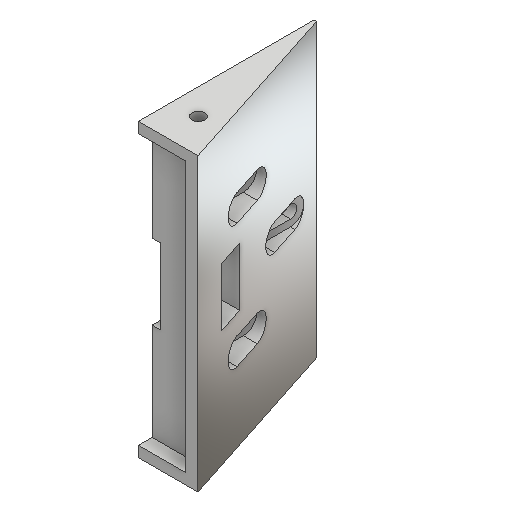
# Autodesk Inventor part: 3DP_PLA_Front_plow
Saved by Autodesk Inventor 2026.1 (Build 301233000, 233)
## iProperties
Created: 2016-05-01
Part Number: 3DP_PLA_Front_plow
Material: Ogólny
Document SubType Name: Modeling
Designer: Andrzej
Density: 1 g/cm^3
Appearance: Domyślna
Mass: 15.1974 g
Surface Area: 84.5843 cm^2
Volume: 15.1974 cm^3
Author: Andrzej
Autodesk Inventor part; units mm, degrees
ref_plane "YZ Plane" through (0, 0, 0) normal (1, 0, 0) x (0, 1, 0)
ref_plane "XZ Plane" through (0, 0, 0) normal (0, 1, 0) x (-1, 0, 0)
ref_plane "XY Plane" through (0, 0, 0) normal (0, 0, 1) x (1, 0, 0)
sketch "Szkic1" plane through (0, 0, 0) normal (0, 0, 1) x (1, 0, 0)
  line L0 (-7.2343, -6.8907) -> (6.6657, -6.8907)
  line L1 (-7.2343, -6.8907) -> (-7.2343, 34.1093)
  line L2 (-7.2343, 34.1093) -> (-6.6343, 34.1093)
  line L3 (-6.6343, 34.1093) -> (6.6657, -6.8907)
  point P0 (0, 0)
  dimension "d0" = 13.9
  dimension "d1" = 41
  dimension "d2" = 0.6
  constraints: 8 end point, 2 horizontal, 1 vertical
  measures "d0" distance of L0.start L0.end
  measures "d1" distance of L0.start L1.end
  measures "d2" distance of L1.end L2.end
extrude "Wyciągnięcie proste1" add sketch "Szkic1" along normal blind 68
sketch "Szkic2" plane through (-7.2343, -6.8907, 0) normal (-1, 0, 0) x (0, 0, 1)
  line L0 (0, 41) -> (0, 0) projected
  line L1 (0, 0) -> (68, 0) projected
  line L2 (68, 41) -> (68, 0) projected
  line L3 (0, 41) -> (68, 41) projected
  line L4 (68, 17.5) -> (68, 0)
  line L5 (53.5, 17.5) -> (68, 17.5)
  line L6 (53.5, 17.5) -> (53.5, 47.1186)
  line L7 (0, 47.1186) -> (53.5, 47.1186)
  line L8 (0, 0) -> (0, 47.1186)
  line L9 (68, 0) -> (0, 0)
  line L10 (68, 0) -> (0, 0)
  line L11 (14.5, 0) -> (14.5, 47.1186)
  line L12 (0, 47.1186) -> (53.5, 47.1186)
  line L13 (14.5, 12) -> (39.4786, 12)
  line L14 (19.5, 13.5) -> (19.5, 20.5) construction
  line L15 (21, 13.5) -> (21, 20.5)
  line L16 (18, 20.5) -> (18, 13.5)
  arc A0 (18, 13.5) -> (21, 13.5) centre (19.5, 13.5) ccw
  arc A1 (21, 20.5) -> (18, 20.5) centre (19.5, 20.5) ccw
  line L17 (48.5, 13.5) -> (48.5, 20.5) construction
  line L18 (50, 13.5) -> (50, 20.5)
  line L19 (47, 20.5) -> (47, 13.5)
  arc A2 (47, 13.5) -> (50, 13.5) centre (48.5, 13.5) ccw
  arc A3 (50, 20.5) -> (47, 20.5) centre (48.5, 20.5) ccw
  line L20 (34, 26.5) -> (34, 33.5) construction
  line L21 (35.5, 26.5) -> (35.5, 33.5)
  line L22 (32.5, 33.5) -> (32.5, 26.5)
  arc A4 (32.5, 26.5) -> (35.5, 26.5) centre (34, 26.5) ccw
  arc A5 (35.5, 33.5) -> (32.5, 33.5) centre (34, 33.5) ccw
  point P0 (0, 6.8907)
  point P1 (82.8727, 0)
  point P2 (19.5, 17)
  point P3 (48.5, 17)
  point P4 (34, 30)
  dimension "d5" = 14.5
  dimension "d6" = 14.5
  dimension "d7" = 12
  dimension "d8" = 5
  dimension "d9" = 5
  dimension "d10" = 5
  dimension "d11" = 5
  dimension "d12" = 18
  dimension "d13" = 19.5
  dimension "d14" = 39
  dimension "d15" = 0
  dimension "d16" = 3.5
  dimension "d17" = 3
  dimension "d18" = 3
  dimension "d19" = 3.5
  dimension "d20" = 3
  constraints: 44 end point, 12 point on circle, 12 tangent, 6 centre point, 5 parallel, 3 midpoint, 3 point on line, 1 horizontal, 1 perpendicular, 1 vertical
  measures "d5" distance between parallel lines of L4 L6
  measures "d6" distance between parallel lines of L8 L11
  measures "d7" distance between parallel lines of L9 L13
  measures "d8" distance from line of L13 point (19.5, 17)
  measures "d9" distance from line of L11 point (19.5, 17)
  measures "d10" distance from line of L13 point (48.5, 17)
  measures "d11" distance from line of L6 point (48.5, 17)
  measures "d12" distance from line of L13 point (34, 30)
  measures "d13" distance from line of L11 point (34, 30)
  measures "d14" distance between parallel lines of L11 L6
  measures "d15" distance between parallel lines of L1 L9
  measures "d16" distance of point (19.5, 17) L14.end
  measures "d17" diameter of A1
  measures "d18" diameter of A3
  measures "d19" distance of point (34, 30) L20.end
  measures "d20" diameter of A5
extrude "Wyciągnięcie proste2" cut sketch "Szkic2" against normal blind 10 contours A0 L16 A1 L15 | A2 L19 A3 L18 | A4 L22 A5 L21
ref_plane "Płaszczyzna konstrukcyjna1" through (4.7657, -6.8907, 0) normal (-1, 0, 0) x (0, 0, 1)
sketch "Szkic3" plane through (4.7657, -6.8907, 0) normal (-1, 0, 0) x (0, 0, 1)
  arc A0 (50, 20.5) -> (47, 20.5) centre (48.5, 20.5) ccw projected
  line L0 (47, 20.5) -> (47, 13.5) projected
  arc A1 (48.7592, 12.0226) -> (50, 13.5) centre (48.5, 13.5) ccw projected
  line L1 (50, 13.5) -> (50, 20.5) projected
  arc A2 (21, 20.5) -> (18, 20.5) centre (19.5, 20.5) ccw projected
  line L2 (18, 20.5) -> (18, 13.5) projected
  arc A3 (19.7592, 12.0226) -> (21, 13.5) centre (19.5, 13.5) ccw projected
  line L3 (21, 13.5) -> (21, 20.5) projected
  arc A4 (35.5, 33.5) -> (32.5, 33.5) centre (34, 33.5) ccw projected
  line L4 (32.5, 33.5) -> (32.5, 26.5) projected
  arc A5 (32.5, 26.5) -> (35.5, 26.5) centre (34, 26.5) ccw projected
  line L5 (35.5, 26.5) -> (35.5, 33.5) projected
  line L6 (0, 0) -> (0, 41) projected
  line L7 (0, 41) -> (68, 41) projected
  line L8 (68, 0) -> (68, 41) projected
  line L9 (0, 0) -> (68, 0) projected
  line L10 (16.4, 13.5) -> (16.4, 20.5)
  arc A6 (22.6, 20.5) -> (16.4, 20.5) centre (19.5, 20.5) ccw
  line L11 (22.6, 20.5) -> (22.6, 13.5)
  arc A7 (16.4, 13.5) -> (22.6, 13.5) centre (19.5, 13.5) ccw
  arc A8 (30.9, 26.5) -> (37.1, 26.5) centre (34, 26.5) ccw
  line L12 (30.9, 26.5) -> (30.9, 33.5)
  arc A9 (37.1, 33.5) -> (30.9, 33.5) centre (34, 33.5) ccw
  line L13 (37.1, 33.5) -> (37.1, 26.5)
  line L14 (45.4, 13.5) -> (45.4, 20.5)
  arc A10 (51.6, 20.5) -> (45.4, 20.5) centre (48.5, 20.5) ccw
  line L15 (51.6, 20.5) -> (51.6, 13.5)
  arc A11 (45.4, 13.5) -> (51.6, 13.5) centre (48.5, 13.5) ccw
  arc A12 (47, 13.5) -> (48.2408, 12.0226) centre (48.5, 13.5) ccw projected
  line L16 (48.2408, 12.0226) -> (48.7592, 12.0226) projected
  arc A13 (18, 13.5) -> (19.2408, 12.0226) centre (19.5, 13.5) ccw projected
  line L17 (19.2408, 12.0226) -> (19.7592, 12.0226) projected
  point P0 (0, 6.8907)
  dimension "d24" = 1.6
  dimension "d25" = 1.6
  dimension "d26" = 1.6
  constraints: 12 end point, 12 point on circle, 6 centre point, 9 other
  measures "d24" distance between parallel lines of L2 L10
  measures "d25" radial gap between concentric circles of A5 A8
  measures "d26" distance between parallel lines of L0 L14
extrude "Wyciągnięcie proste3" cut sketch "Szkic3" along normal blind 8 contours L10 A6 L11 A7 | L14 A10 L15 A11
extrude "Wyciągnięcie proste4" cut sketch "Szkic3" along normal blind 10 contours L12 A9 L13 A8
sketch "Szkic4" plane through (-7.2343, -6.8907, 0) normal (0, -1, 0) x (1, 0, 0)
  line L0 (0, 0) -> (13.9, 0) projected
  line L1 (13.9, 0) -> (13.9, 68) projected
  line L2 (0, 68) -> (13.9, 68) projected
  line L3 (0, 0) -> (0, 68) projected
  line L4 (0, 0) -> (0, 68) projected
  line L5 (0, 65.5) -> (10.9, 65.5)
  line L6 (10.9, 65.5) -> (10.9, 2.5)
  line L7 (10.9, 2.5) -> (0, 2.5)
  point P0 (7.2343, 0)
  dimension "d31" = 2.5
  dimension "d32" = 3
  dimension "d33" = 2.5
  constraints: 6 end point, 3 perpendicular, 2 point on line
  measures "d31" distance between parallel lines of L2 L5
  measures "d32" distance between parallel lines of L1 L6
  measures "d33" distance between parallel lines of L0 L7
extrude "Wyciągnięcie proste5" cut sketch "Szkic4" against normal blind 3.2 contours L3 L5 L6 L7
sketch "Szkic5" plane through (-7.2343, -6.8907, 0) normal (-1, 0, 0) x (0, 0, 1)
  line L0 (2.5, 0) -> (2.5, 3.2) projected
  line L1 (2.5, 3.2) -> (65.5, 3.2) projected
  line L2 (65.5, 3.2) -> (65.5, 0) projected
  line L3 (65.5, 0) -> (68, 0) projected
  line L4 (68, 41) -> (68, 0) projected
  line L5 (0, 41) -> (68, 41) projected
  line L6 (0, 41) -> (0, 0) projected
  line L7 (0, 0) -> (2.5, 0) projected
  arc A0 (35.5, 33.5) -> (32.5, 33.5) centre (34, 33.5) ccw projected
  line L8 (35.5, 33.5) -> (35.5, 26.5) projected
  arc A1 (32.5, 26.5) -> (35.5, 26.5) centre (34, 26.5) ccw projected
  line L9 (32.5, 26.5) -> (32.5, 33.5) projected
  arc A2 (21, 20.5) -> (18, 20.5) centre (19.5, 20.5) ccw projected
  line L10 (21, 20.5) -> (21, 13.5) projected
  arc A3 (18, 13.5) -> (21, 13.5) centre (19.5, 13.5) ccw projected
  line L11 (18, 13.5) -> (18, 20.5) projected
  arc A4 (50, 20.5) -> (47, 20.5) centre (48.5, 20.5) ccw projected
  line L12 (50, 20.5) -> (50, 13.5) projected
  arc A5 (47, 13.5) -> (50, 13.5) centre (48.5, 13.5) ccw projected
  line L13 (47, 13.5) -> (47, 20.5) projected
  line L14 (65.5, 3.2) -> (2.5, 3.2) projected
  line L15 (29, 3.2) -> (39, 3.2)
  line L16 (39, 3.2) -> (39, 21.2)
  line L17 (39, 21.2) -> (29, 21.2)
  line L18 (29, 21.2) -> (29, 3.2)
  line L19 (2.5, 3.2) -> (65.5, 3.2) projected
  point P0 (0, 6.8907)
  dimension "d36" = 68
  dimension "d37" = 10
  dimension "d38" = 29
  dimension "d39" = 18
  constraints: 8 end point, 2 parallel, 1 horizontal, 1 perpendicular, 1 point on line
  measures "d36" distance of L5.start L4.start
  measures "d37" distance between parallel lines of L16 L18
  measures "d38" distance between parallel lines of L6 L18
  measures "d39" distance between parallel lines of L1 L17
extrude "Wyciągnięcie proste6" cut sketch "Szkic5" against normal blind 2 contours L18 L17 L16 L1
sketch "Szkic6" plane through (-7.2343, -6.8907, 0) normal (-1, 0, 0) x (0, 0, 1)
  line L0 (39, 21.2) -> (39, 3.2) projected
  line L1 (39, 3.2) -> (65.5, 3.2) projected
  line L2 (65.5, 3.2) -> (65.5, 0) projected
  line L3 (65.5, 0) -> (68, 0) projected
  line L4 (68, 41) -> (68, 0) projected
  line L5 (0, 41) -> (68, 41) projected
  line L6 (0, 41) -> (0, 0) projected
  line L7 (0, 0) -> (2.5, 0) projected
  line L8 (2.5, 0) -> (2.5, 3.2) projected
  line L9 (2.5, 3.2) -> (29, 3.2) projected
  line L10 (29, 3.2) -> (29, 21.2) projected
  line L11 (29, 21.2) -> (39, 21.2) projected
  arc A0 (35.5, 33.5) -> (32.5, 33.5) centre (34, 33.5) ccw projected
  line L12 (35.5, 33.5) -> (35.5, 26.5) projected
  arc A1 (32.5, 26.5) -> (35.5, 26.5) centre (34, 26.5) ccw projected
  line L13 (32.5, 26.5) -> (32.5, 33.5) projected
  arc A2 (21, 20.5) -> (18, 20.5) centre (19.5, 20.5) ccw projected
  line L14 (21, 20.5) -> (21, 13.5) projected
  arc A3 (18, 13.5) -> (21, 13.5) centre (19.5, 13.5) ccw projected
  line L15 (18, 13.5) -> (18, 20.5) projected
  arc A4 (50, 20.5) -> (47, 20.5) centre (48.5, 20.5) ccw projected
  line L16 (50, 20.5) -> (50, 13.5) projected
  arc A5 (47, 13.5) -> (50, 13.5) centre (48.5, 13.5) ccw projected
  line L17 (47, 13.5) -> (47, 20.5) projected
  line L18 (27.2, 14.4) -> (40.8, 14.4)
  line L19 (40.8, 14.4) -> (40.8, 8.2)
  line L20 (40.8, 8.2) -> (27.2, 8.2)
  line L21 (27.2, 8.2) -> (27.2, 14.4)
  line L22 (40.8, 14.8) -> (27.2, 14.8)
  line L23 (27.2, 7.8) -> (40.8, 7.8)
  line L24 (27.2, 14.4) -> (27.2, 14.8)
  line L25 (27.2, 8.2) -> (27.2, 7.8)
  line L26 (40.8, 8.2) -> (40.8, 7.8)
  line L27 (40.8, 14.4) -> (40.8, 14.8)
  point P0 (0, 6.8907)
  dimension "d47" = 13.6
  dimension "d48" = 6.2
  dimension "d49" = 68
  dimension "d50" = 27.2
  dimension "d51" = 5
  dimension "d54" = 0.4
  dimension "d61" = 0.4
  constraints: 20 end point, 4 parallel, 3 perpendicular, 1 horizontal, 1 point on line
  measures "d47" distance of L19.end L20.end
  measures "d48" distance of L20.end L18.start
  measures "d49" distance between parallel lines of L4 L6
  measures "d50" distance between parallel lines of L6 L21
  measures "d51" distance between parallel lines of L9 L20
  measures "d54" distance between parallel lines of L18 L22
  measures "d61" distance between parallel lines of L20 L23
extrude "Wyciągnięcie proste7" cut sketch "Szkic6" against normal through all contours L18 L19 L20 L0 | L0 L20 L10 L18 | L10 L20 L21 L18
extrude "Wyciągnięcie proste8" cut sketch "Szkic6" against normal blind 4.8 contours L22 L27 L18 L0 | L0 L18 L10 L22 | L10 L18 L24 L22 | L20 L26 L23 L0 | L0 L23 L10 L20 | L10 L23 L25 L20
sketch "Szkic7" plane through (-7.2343, -6.8907, 0) normal (-1, 0, 0) x (0, 0, 1)
  line L0 (40.8, 7.8) -> (39, 7.8) projected
  line L1 (39, 7.8) -> (39, 3.2) projected
  line L2 (39, 3.2) -> (65.5, 3.2) projected
  line L3 (65.5, 3.2) -> (65.5, 0) projected
  line L4 (65.5, 0) -> (68, 0) projected
  line L5 (68, 41) -> (68, 0) projected
  line L6 (0, 41) -> (68, 41) projected
  line L7 (0, 41) -> (0, 0) projected
  line L8 (0, 0) -> (2.5, 0) projected
  line L9 (2.5, 0) -> (2.5, 3.2) projected
  line L10 (2.5, 3.2) -> (29, 3.2) projected
  line L11 (29, 3.2) -> (29, 7.8) projected
  line L12 (29, 7.8) -> (27.2, 7.8) projected
  line L13 (27.2, 7.8) -> (27.2, 14.8) projected
  line L14 (27.2, 14.8) -> (29, 14.8) projected
  line L15 (29, 14.8) -> (29, 21.2) projected
  line L16 (29, 21.2) -> (39, 21.2) projected
  line L17 (39, 21.2) -> (39, 14.8) projected
  line L18 (39, 14.8) -> (40.8, 14.8) projected
  line L19 (40.8, 14.8) -> (40.8, 7.8) projected
  arc A0 (35.5, 33.5) -> (32.5, 33.5) centre (34, 33.5) ccw projected
  line L20 (35.5, 33.5) -> (35.5, 26.5) projected
  arc A1 (32.5, 26.5) -> (35.5, 26.5) centre (34, 26.5) ccw projected
  line L21 (32.5, 26.5) -> (32.5, 33.5) projected
  arc A2 (21, 20.5) -> (18, 20.5) centre (19.5, 20.5) ccw projected
  line L22 (21, 20.5) -> (21, 13.5) projected
  arc A3 (18, 13.5) -> (21, 13.5) centre (19.5, 13.5) ccw projected
  line L23 (18, 13.5) -> (18, 20.5) projected
  arc A4 (50, 20.5) -> (47, 20.5) centre (48.5, 20.5) ccw projected
  line L24 (50, 20.5) -> (50, 13.5) projected
  arc A5 (47, 13.5) -> (50, 13.5) centre (48.5, 13.5) ccw projected
  line L25 (47, 13.5) -> (47, 20.5) projected
  line L26 (29, 14.8) -> (39, 14.8) projected
  line L27 (39, 7.8) -> (29, 7.8) projected
  line L28 (27.2, 14.8) -> (40.8, 14.8)
  line L29 (40.8, 14.8) -> (40.8, 7.8)
  line L30 (40.8, 7.8) -> (27.2, 7.8)
  line L31 (27.2, 7.8) -> (27.2, 14.8)
  line L32 (25.2, 16.8) -> (42.8, 16.8)
  line L33 (42.8, 16.8) -> (42.8, 5.8)
  line L34 (25.2, 5.8) -> (25.2, 16.8)
  line L35 (25.2, 5.8) -> (25.2, 3.2)
  line L36 (42.8, 5.8) -> (42.8, 3.2)
  line L37 (39, 3.2) -> (65.5, 3.2) projected
  line L38 (25.2, 3.2) -> (42.8, 3.2)
  point P0 (0, 6.8907)
  dimension "d57" = 2
  constraints: 20 end point, 4 parallel, 3 perpendicular, 2 point on line, 1 collinear, 1 horizontal, 1 other
  measures "d57" distance between parallel lines of L31 L34
extrude "Wyciągnięcie proste9" cut sketch "Szkic7" against normal blind 2 contours L19 L18 L17 L32 L33 L36 L2 L1 L0 | L1 L38 L11 L27 | L11 L10 L35 L34 L32 L15 L14 L13 L12 | L26 L15 L32 L17
fillet "Zaokrąglenie1" radius 2 4 edges at (-6.2343, 9.9093, 29) (-6.2343, 9.9093, 39) (-6.2343, 9.9093, 25.2) (-6.2343, 9.9093, 42.8)
sketch "Szkic8" plane through (0, 0, 0) normal (0, 0, -1) x (-1, 0, 0)
  line L0 (7.2343, -6.8907) -> (-6.6657, -6.8907) projected
  line L1 (7.2343, 34.1093) -> (7.2343, -6.8907) projected
  line L2 (6.6343, 34.1093) -> (7.2343, 34.1093) projected
  line L3 (-6.6657, -6.8907) -> (6.6343, 34.1093) projected
  circle A0 centre (1.2343, 1.1093) radius 5
  circle A1 centre (1.2343, 1.1093) radius 1.5
  point P0 (0, 0)
  dimension "d62" = 8
  dimension "d63" = 10
  dimension "d64" = 6
  dimension "d65" = 3
  constraints: 2 centre point, 2 coincident
  measures "d62" distance from line of L0 point (1.234, 1.109)
  measures "d63" diameter of A0
  measures "d64" distance from line of L1 A0.centre
  measures "d65" diameter of A1
extrude "Wyciągnięcie proste10" cut sketch "Szkic8" against normal blind 10 contours A1
sketch "Szkic9" plane through (0, 0, 68) normal (0, 0, 1) x (1, 0, 0)
  line L0 (-7.2343, -6.8907) -> (6.6657, -6.8907) projected
  line L1 (6.6657, -6.8907) -> (-6.6343, 34.1093) projected
  line L2 (-6.6343, 34.1093) -> (-7.2343, 34.1093) projected
  line L3 (-7.2343, 34.1093) -> (-7.2343, -6.8907) projected
  circle A0 centre (-1.2343, 1.1093) radius 1.5 projected
  point P0 (0, 0)
extrude "Wyciągnięcie proste11" cut sketch "Szkic9" against normal blind 10 contours A0
sketch "Szkic10" plane through (-7.2343, -6.8907, 0) normal (-1, 0, 0) x (0, 0, 1)
  line L0 (10, 6.5) -> (10, 9.5) projected
  line L1 (58, 9.5) -> (58, 6.5) projected
  line L2 (0, 9.5) -> (10, 9.5) projected
  line L3 (0, 6.5) -> (10, 6.5) projected
  line L4 (68, 6.5) -> (58, 6.5) projected
  line L5 (68, 9.5) -> (58, 9.5) projected
  line L6 (7, 11) -> (10, 11)
  line L7 (10, 11) -> (10, 5)
  line L8 (10, 5) -> (7, 5)
  line L9 (7, 5) -> (7, 11)
  line L10 (58, 5) -> (61, 5)
  line L11 (61, 5) -> (61, 11)
  line L12 (61, 11) -> (58, 11)
  line L13 (58, 11) -> (58, 5)
  point P0 (0, 6.8907)
  dimension "d70" = 3
  dimension "d71" = 6
  dimension "d72" = 0
  dimension "d73" = 1.5
  dimension "d74" = 3
  dimension "d75" = 3
  dimension "d76" = 6
  dimension "d77" = 1.5
  constraints: 16 end point, 4 parallel, 2 horizontal, 2 perpendicular
  measures "d70" distance of L7.end L8.end
  measures "d71" distance of L6.end L7.end
  measures "d72" distance between parallel lines of L0 L7
  measures "d73" distance between parallel lines of L6 L2
  measures "d74" distance between parallel lines of L2 L3
  measures "d75" distance of L12.end L11.end
  measures "d76" distance of L11.end L10.end
  measures "d77" distance between parallel lines of L12 L5
extrude "Wyciągnięcie proste12" cut sketch "Szkic10" against normal blind 9.5
equation "\"d6\" = d5"
equation "\"d9\" = d8"
equation "\"d10\" = d8"
equation "\"d11\" = d8"
equation "\"d13\" = 0.5 * d14"
equation "\"d38\" = -0.5 * d37 + 0.5 * d36"
equation "\"d50\" = -0.5 * d47 + 0.5 * d49"
equation "\"d61\" = d54"
equation "\"d73\" = -0.5 * d74 + 0.5 * d71"
equation "\"d77\" = d73"
